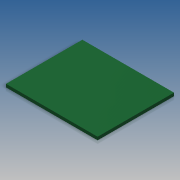
# Autodesk Inventor part: 97622-PCB
Saved by Autodesk Inventor 2016 SP2 (Build 200236200, 236)
## iProperties
Created: 2015-08-21
Part Number: 97622-PCB
Material: ABS Plastic
Document SubType Name: Modeling
Designer: D. Kohfeld
Density: 1.06 g/cm^3
Appearance: PCB
Mass: 3.25632 g
Surface Area: 41.216 cm^2
Volume: 3.072 cm^3
Author: D. Kohfeld
Autodesk Inventor part; units mm, degrees
ref_plane "YZ Plane" through (0, 0, 0) normal (1, 0, 0) x (0, 1, 0)
ref_plane "XZ Plane" through (0, 0, 0) normal (0, 1, 0) x (-1, 0, 0)
ref_plane "XY Plane" through (0, 0, 0) normal (0, 0, 1) x (1, 0, 0)
sketch "Sketch2" plane through (0, 0, 0) normal (0, 1, 0) x (-1, 0, 0)
  line L0 (-24, 20) -> (24, 20)
  line L1 (24, 20) -> (24, -20)
  line L2 (24, -20) -> (-24, -20)
  line L3 (-24, -20) -> (-24, 20)
  point P0 (0, 0)
  point P1 (0, 20)
  point P2 (-24, 0)
  dimension "d0" = 40
  dimension "d1" = 48
  constraints: 8 end point, 2 midpoint, 2 parallel, 1 horizontal, 1 horizontal alignment, 1 perpendicular, 1 vertical alignment
  measures "d0" distance of L2.end L0.start
  measures "d1" distance of L0.start L0.end
extrude "Extrusion1" add sketch "Sketch2" along normal mid plane 1.6
equation "\"d2\" = wall"
equation "\"wall\" = 1.6"
body "Solid1"
